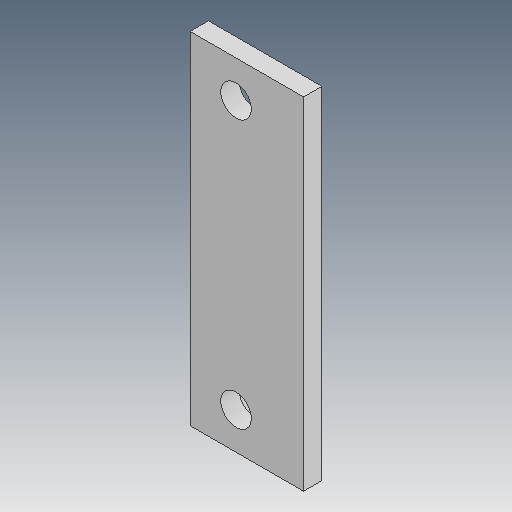
# Autodesk Inventor part: pulley_tab_right_A
Saved by Autodesk Inventor 2025.2 (Build 292293000, 293)
## iProperties
Created: 2025-02-16
Part Number: pulley_tab_right_A
Material: Generic
Document SubType Name: Modeling
Designer: email
Density: 1 g/cm^3
Appearance: Default
Author: email
Autodesk Inventor part; units mm, degrees
ref_plane "YZ Plane" through (0, 0, 0) normal (1, 0, 0) x (0, 1, 0)
ref_plane "XZ Plane" through (0, 0, 0) normal (0, 1, 0) x (-1, 0, 0)
ref_plane "XY Plane" through (0, 0, 0) normal (0, 0, 1) x (1, 0, 0)
sketch "Sketch1" plane through (0, 0, 0) normal (0, 0, 1) x (1, 0, 0)
  line L0 (0, 0) -> (18.5, 0)
  line L1 (18.5, 0) -> (18.5, 55.67)
  line L2 (18.5, 55.67) -> (0, 55.67)
  line L3 (0, 55.67) -> (0, 0)
  circle A0 centre (7.5, 6) radius 2.5
  circle A1 centre (7.5, 49.67) radius 2.5
  point P0 (9.25, 55.67)
  dimension "d0" = 18.5
  dimension "d1" = 55.67
  dimension "d2" = 5
  dimension "d3" = 11
  dimension "d4" = 6
  dimension "d5" = 6
  dimension "d6" = 11
  constraints: 8 end point, 2 centre point, 2 parallel, 1 equal radius, 1 horizontal, 1 midpoint, 1 perpendicular
  measures "d0" distance of L1.end L2.end
  measures "d1" distance of L0.end L1.end
  measures "d2" diameter of A0
  measures "d3" distance from line of L1 A0.centre
  measures "d4" distance from line of L0 A0.centre
  measures "d5" vertical distance of point (9.25, 55.67) A1.centre
  measures "d6" distance from line of L1 A1.centre
extrude "Extrusion1" add sketch "Sketch1" along normal blind 3
body "Solid1"
